Autodesk Inventor part; units mm, degrees
(part 2 of 2)
  spline S217 degree 2 poles (-59.869, -3.174) (-59.9555, -3.2654) (-60.0444, -3.4852) (-60.0567, -3.6309) knots 0 0 0 1 2 2 2
  line L196 (-60.0567, -3.6309) -> (-58.8489, -3.6309)
  line L197 (-54.9784, -5.029) -> (-56.7444, -5.029)
  line L198 (-56.7444, -5.029) -> (-56.7444, -1.981)
  line L199 (-56.7444, -1.981) -> (-56.3394, -1.981)
  line L200 (-56.3394, -1.981) -> (-56.3394, -4.6683)
  line L201 (-56.3394, -4.6683) -> (-54.9784, -4.6683)
  line L202 (-54.9784, -4.6683) -> (-54.9784, -5.029)
  spline S218 degree 2 poles (-53.6964, -5.0808) (-54.2448, -5.0808) (-54.8475, -4.4658) (-54.8475, -3.8977) knots 0 0 0 1 2 2 2
  spline S219 degree 2 poles (-54.8475, -3.8977) (-54.8475, -3.3395) (-54.2621, -2.6775) (-53.7903, -2.6775) knots 0 0 0 1 2 2 2
  spline S220 degree 2 poles (-53.7903, -2.6775) (-53.5779, -2.6775) (-53.2494, -2.801) (-53.1283, -2.9319) knots 0 0 0 1 2 2 2
  spline S221 degree 2 poles (-53.1283, -2.9319) (-53.0048, -3.0628) (-52.8739, -3.4407) (-52.8739, -3.7149) knots 0 0 0 1 2 2 2
  line L203 (-52.8739, -3.7149) -> (-52.8739, -3.9249)
  line L204 (-52.8739, -3.9249) -> (-54.4572, -3.9249)
  spline S222 degree 2 poles (-54.4572, -3.9249) (-54.4572, -4.3225) (-54.0571, -4.7449) (-53.7014, -4.7449) knots 0 0 0 1 2 2 2
  spline S223 degree 2 poles (-53.7014, -4.7449) (-53.5754, -4.7449) (-53.3309, -4.6881) (-53.2321, -4.6436) knots 0 0 0 1 2 2 2
  spline S224 degree 2 poles (-53.2321, -4.6436) (-53.1283, -4.5942) (-52.9851, -4.5078) (-52.9381, -4.4683) knots 0 0 0 1 2 2 2
  line L205 (-52.9381, -4.4683) -> (-52.9159, -4.4683)
  line L206 (-52.9159, -4.4683) -> (-52.9159, -4.8882)
  spline S225 degree 2 poles (-52.9159, -4.8882) (-52.9826, -4.9153) (-53.1851, -4.9944) (-53.2642, -5.0166) knots 0 0 0 1 2 2 2
  spline S226 degree 2 poles (-53.2642, -5.0166) (-53.3753, -5.0487) (-53.5581, -5.0808) (-53.6964, -5.0808) knots 0 0 0 1 2 2 2
  spline S227 degree 2 poles (-53.2494, -3.6309) (-53.2543, -3.4753) (-53.3185, -3.2481) (-53.3803, -3.1715) knots 0 0 0 1 2 2 2
  spline S228 degree 2 poles (-53.3803, -3.1715) (-53.447, -3.085) (-53.6569, -2.9937) (-53.8125, -2.9937) knots 0 0 0 1 2 2 2
  spline S229 degree 2 poles (-53.8125, -2.9937) (-53.9657, -2.9937) (-54.1806, -3.085) (-54.2695, -3.174) knots 0 0 0 1 2 2 2
  spline S230 degree 2 poles (-54.2695, -3.174) (-54.3559, -3.2654) (-54.4449, -3.4852) (-54.4572, -3.6309) knots 0 0 0 1 2 2 2
  line L207 (-54.4572, -3.6309) -> (-53.2494, -3.6309)
  line L208 (-49.8901, -5.029) -> (-49.8901, -3.705)
  spline S231 degree 2 poles (-49.8901, -3.705) (-49.8901, -3.5469) (-49.9148, -3.2777) (-49.9544, -3.2036) knots 0 0 0 1 2 2 2
  spline S232 degree 2 poles (-49.9544, -3.2036) (-49.9939, -3.1221) (-50.1446, -3.0431) (-50.2755, -3.0431) knots 0 0 0 1 2 2 2
  spline S233 degree 2 poles (-50.2755, -3.0431) (-50.394, -3.0431) (-50.6657, -3.1888) (-50.809, -3.3271) knots 0 0 0 1 2 2 2
  spline S234 degree 2 poles (-50.809, -3.3271) (-50.8065, -3.3617) (-50.8016, -3.458) (-50.8016, -3.5222) knots 0 0 0 1 2 2 2
  line L209 (-50.8016, -3.5222) -> (-50.8016, -5.029)
  line L210 (-50.8016, -5.029) -> (-51.1869, -5.029)
  line L211 (-51.1869, -5.029) -> (-51.1869, -3.705)
  spline S235 degree 2 poles (-51.1869, -3.705) (-51.1869, -3.5469) (-51.2116, -3.2777) (-51.2511, -3.2036) knots 0 0 0 1 2 2 2
  spline S236 degree 2 poles (-51.2511, -3.2036) (-51.2906, -3.1221) (-51.4413, -3.0431) (-51.5722, -3.0431) knots 0 0 0 1 2 2 2
  spline S237 degree 2 poles (-51.5722, -3.0431) (-51.6957, -3.0431) (-51.9699, -3.1987) (-52.0983, -3.3197) knots 0 0 0 1 2 2 2
  line L212 (-52.0983, -3.3197) -> (-52.0983, -5.029)
  line L213 (-52.0983, -5.029) -> (-52.4837, -5.029)
  line L214 (-52.4837, -5.029) -> (-52.4837, -2.7417)
  line L215 (-52.4837, -2.7417) -> (-52.0983, -2.7417)
  line L216 (-52.0983, -2.7417) -> (-52.0983, -2.9937)
  spline S238 degree 2 poles (-52.0983, -2.9937) (-51.9477, -2.843) (-51.6513, -2.6775) (-51.4734, -2.6775) knots 0 0 0 1 2 2 2
  spline S239 degree 2 poles (-51.4734, -2.6775) (-51.2709, -2.6775) (-50.9572, -2.8627) (-50.8757, -3.0727) knots 0 0 0 1 2 2 2
  spline S240 degree 2 poles (-50.8757, -3.0727) (-50.7003, -2.8776) (-50.3693, -2.6775) (-50.1767, -2.6775) knots 0 0 0 1 2 2 2
  spline S241 degree 2 poles (-50.1767, -2.6775) (-50.0285, -2.6775) (-49.7864, -2.7689) (-49.6975, -2.8726) knots 0 0 0 1 2 2 2
  spline S242 degree 2 poles (-49.6975, -2.8726) (-49.6061, -2.9764) (-49.5048, -3.2876) (-49.5048, -3.5222) knots 0 0 0 1 2 2 2
  line L217 (-49.5048, -3.5222) -> (-49.5048, -5.029)
  line L218 (-49.5048, -5.029) -> (-49.8901, -5.029)
  spline S243 degree 2 poles (-47.0472, -3.8483) (-47.0472, -4.409) (-47.5906, -5.0932) (-48.0006, -5.0932) knots 0 0 0 1 2 2 2
  spline S244 degree 2 poles (-48.0006, -5.0932) (-48.1858, -5.0932) (-48.4501, -5.0018) (-48.5786, -4.9227) knots 0 0 0 1 2 2 2
  line L219 (-48.5786, -4.9227) -> (-48.6033, -5.029)
  line L220 (-48.6033, -5.029) -> (-48.9639, -5.029)
  line L221 (-48.9639, -5.029) -> (-48.9639, -1.8451)
  line L222 (-48.9639, -1.8451) -> (-48.5786, -1.8451)
  line L223 (-48.5786, -1.8451) -> (-48.5786, -2.9813)
  spline S245 degree 2 poles (-48.5786, -2.9813) (-48.4328, -2.8504) (-48.0944, -2.6775) (-47.8796, -2.6775) knots 0 0 0 1 2 2 2
  spline S246 degree 2 poles (-47.8796, -2.6775) (-47.4918, -2.6775) (-47.0472, -3.2975) (-47.0472, -3.8483) knots 0 0 0 1 2 2 2
  spline S247 degree 2 poles (-47.4448, -3.8779) (-47.4448, -3.4679) (-47.6943, -3.0431) (-47.9709, -3.0431) knots 0 0 0 1 2 2 2
  spline S248 degree 2 poles (-47.9709, -3.0431) (-48.1266, -3.0431) (-48.4477, -3.1913) (-48.5786, -3.3049) knots 0 0 0 1 2 2 2
  line L224 (-48.5786, -3.3049) -> (-48.5786, -4.6165)
  spline S249 degree 2 poles (-48.5786, -4.6165) (-48.4328, -4.6881) (-48.2081, -4.7474) (-48.0747, -4.7474) knots 0 0 0 1 2 2 2
  spline S250 degree 2 poles (-48.0747, -4.7474) (-47.7808, -4.7474) (-47.4448, -4.3299) (-47.4448, -3.8779) knots 0 0 0 1 2 2 2
  spline S251 degree 2 poles (-44.7673, -3.8853) (-44.7673, -4.4633) (-45.3231, -5.0932) (-45.7874, -5.0932) knots 0 0 0 1 2 2 2
  spline S252 degree 2 poles (-45.7874, -5.0932) (-46.2642, -5.0932) (-46.81, -4.4436) (-46.81, -3.8853) knots 0 0 0 1 2 2 2
  spline S253 degree 2 poles (-46.81, -3.8853) (-46.81, -3.3123) (-46.2469, -2.6775) (-45.7874, -2.6775) knots 0 0 0 1 2 2 2
  spline S254 degree 2 poles (-45.7874, -2.6775) (-45.3231, -2.6775) (-44.7673, -3.3098) (-44.7673, -3.8853) knots 0 0 0 1 2 2 2
  spline S255 degree 2 poles (-45.165, -3.8853) (-45.165, -3.4407) (-45.4886, -3.0085) (-45.7874, -3.0085) knots 0 0 0 1 2 2 2
  spline S256 degree 2 poles (-45.7874, -3.0085) (-46.0863, -3.0085) (-46.4124, -3.4407) (-46.4124, -3.8853) knots 0 0 0 1 2 2 2
  spline S257 degree 2 poles (-46.4124, -3.8853) (-46.4124, -4.3176) (-46.0863, -4.7622) (-45.7874, -4.7622) knots 0 0 0 1 2 2 2
  spline S258 degree 2 poles (-45.7874, -4.7622) (-45.491, -4.7622) (-45.165, -4.325) (-45.165, -3.8853) knots 0 0 0 1 2 2 2
  line L225 (-42.0034, -3.8804) -> (-43.1569, -3.8804)
  line L226 (-43.1569, -3.8804) -> (-43.1569, -3.5099)
  line L227 (-43.1569, -3.5099) -> (-42.0034, -3.5099)
  line L228 (-42.0034, -3.5099) -> (-42.0034, -3.8804)
  line L229 (-39.4914, -5.029) -> (-39.4914, -2.3416)
  line L230 (-39.4914, -2.3416) -> (-40.514, -2.3416)
  line L231 (-40.514, -2.3416) -> (-40.514, -1.981)
  line L232 (-40.514, -1.981) -> (-38.0637, -1.981)
  line L233 (-38.0637, -1.981) -> (-38.0637, -2.3416)
  line L234 (-38.0637, -2.3416) -> (-39.0863, -2.3416)
  line L235 (-39.0863, -2.3416) -> (-39.0863, -5.029)
  line L236 (-39.0863, -5.029) -> (-39.4914, -5.029)
  spline S259 degree 2 poles (-35.9049, -3.8853) (-35.9049, -4.4633) (-36.4607, -5.0932) (-36.925, -5.0932) knots 0 0 0 1 2 2 2
  spline S260 degree 2 poles (-36.925, -5.0932) (-37.4017, -5.0932) (-37.9476, -4.4436) (-37.9476, -3.8853) knots 0 0 0 1 2 2 2
  spline S261 degree 2 poles (-37.9476, -3.8853) (-37.9476, -3.3123) (-37.3845, -2.6775) (-36.925, -2.6775) knots 0 0 0 1 2 2 2
  spline S262 degree 2 poles (-36.925, -2.6775) (-36.4607, -2.6775) (-35.9049, -3.3098) (-35.9049, -3.8853) knots 0 0 0 1 2 2 2
  spline S263 degree 2 poles (-36.3026, -3.8853) (-36.3026, -3.4407) (-36.6262, -3.0085) (-36.925, -3.0085) knots 0 0 0 1 2 2 2
  spline S264 degree 2 poles (-36.925, -3.0085) (-37.2239, -3.0085) (-37.5499, -3.4407) (-37.5499, -3.8853) knots 0 0 0 1 2 2 2
  spline S265 degree 2 poles (-37.5499, -3.8853) (-37.5499, -4.3176) (-37.2239, -4.7622) (-36.925, -4.7622) knots 0 0 0 1 2 2 2
  spline S266 degree 2 poles (-36.925, -4.7622) (-36.6286, -4.7622) (-36.3026, -4.325) (-36.3026, -3.8853) knots 0 0 0 1 2 2 2
  line L237 (-32.9162, -5.029) -> (-32.9162, -3.705)
  spline S267 degree 2 poles (-32.9162, -3.705) (-32.9162, -3.5469) (-32.9409, -3.2777) (-32.9804, -3.2036) knots 0 0 0 1 2 2 2
  spline S268 degree 2 poles (-32.9804, -3.2036) (-33.0199, -3.1221) (-33.1706, -3.0431) (-33.3015, -3.0431) knots 0 0 0 1 2 2 2
  spline S269 degree 2 poles (-33.3015, -3.0431) (-33.4201, -3.0431) (-33.6918, -3.1888) (-33.835, -3.3271) knots 0 0 0 1 2 2 2
  spline S270 degree 2 poles (-33.835, -3.3271) (-33.8326, -3.3617) (-33.8276, -3.458) (-33.8276, -3.5222) knots 0 0 0 1 2 2 2
  line L238 (-33.8276, -3.5222) -> (-33.8276, -5.029)
  line L239 (-33.8276, -5.029) -> (-34.213, -5.029)
  line L240 (-34.213, -5.029) -> (-34.213, -3.705)
  spline S271 degree 2 poles (-34.213, -3.705) (-34.213, -3.5469) (-34.2377, -3.2777) (-34.2772, -3.2036) knots 0 0 0 1 2 2 2
  spline S272 degree 2 poles (-34.2772, -3.2036) (-34.3167, -3.1221) (-34.4674, -3.0431) (-34.5983, -3.0431) knots 0 0 0 1 2 2 2
  spline S273 degree 2 poles (-34.5983, -3.0431) (-34.7218, -3.0431) (-34.9959, -3.1987) (-35.1244, -3.3197) knots 0 0 0 1 2 2 2
  line L241 (-35.1244, -3.3197) -> (-35.1244, -5.029)
  line L242 (-35.1244, -5.029) -> (-35.5097, -5.029)
  line L243 (-35.5097, -5.029) -> (-35.5097, -2.7417)
  line L244 (-35.5097, -2.7417) -> (-35.1244, -2.7417)
  line L245 (-35.1244, -2.7417) -> (-35.1244, -2.9937)
  spline S274 degree 2 poles (-35.1244, -2.9937) (-34.9737, -2.843) (-34.6773, -2.6775) (-34.4995, -2.6775) knots 0 0 0 1 2 2 2
  spline S275 degree 2 poles (-34.4995, -2.6775) (-34.2969, -2.6775) (-33.9832, -2.8627) (-33.9017, -3.0727) knots 0 0 0 1 2 2 2
  spline S276 degree 2 poles (-33.9017, -3.0727) (-33.7264, -2.8776) (-33.3954, -2.6775) (-33.2027, -2.6775) knots 0 0 0 1 2 2 2
  spline S277 degree 2 poles (-33.2027, -2.6775) (-33.0545, -2.6775) (-32.8125, -2.7689) (-32.7235, -2.8726) knots 0 0 0 1 2 2 2
  spline S278 degree 2 poles (-32.7235, -2.8726) (-32.6321, -2.9764) (-32.5309, -3.2876) (-32.5309, -3.5222) knots 0 0 0 1 2 2 2
  line L246 (-32.5309, -3.5222) -> (-32.5309, -5.029)
  line L247 (-32.5309, -5.029) -> (-32.9162, -5.029)
  spline S279 degree 2 poles (-28.7246, -2.8998) (-28.7246, -3.0974) (-28.8654, -3.4531) (-28.9913, -3.5766) knots 0 0 0 1 2 2 2
  spline S280 degree 2 poles (-28.9913, -3.5766) (-29.1494, -3.7322) (-29.5767, -3.8927) (-29.9028, -3.8927) knots 0 0 0 1 2 2 2
  line L248 (-29.9028, -3.8927) -> (-30.2461, -3.8927)
  line L249 (-30.2461, -3.8927) -> (-30.2461, -5.029)
  line L250 (-30.2461, -5.029) -> (-30.6512, -5.029)
  line L251 (-30.6512, -5.029) -> (-30.6512, -1.981)
  line L252 (-30.6512, -1.981) -> (-29.8855, -1.981)
  spline S281 degree 2 poles (-29.8855, -1.981) (-29.6138, -1.981) (-29.2334, -2.0699) (-29.0877, -2.1711) knots 0 0 0 1 2 2 2
  spline S282 degree 2 poles (-29.0877, -2.1711) (-28.9172, -2.2872) (-28.7246, -2.6454) (-28.7246, -2.8998) knots 0 0 0 1 2 2 2
  spline S283 degree 2 poles (-29.1469, -2.9121) (-29.1469, -2.7541) (-29.2556, -2.5219) (-29.3668, -2.4478) knots 0 0 0 1 2 2 2
  spline S284 degree 2 poles (-29.3668, -2.4478) (-29.4631, -2.3836) (-29.72, -2.3317) (-29.9102, -2.3317) knots 0 0 0 1 2 2 2
  line L253 (-29.9102, -2.3317) -> (-30.2461, -2.3317)
  line L254 (-30.2461, -2.3317) -> (-30.2461, -3.5469)
  line L255 (-30.2461, -3.5469) -> (-29.9695, -3.5469)
  spline S285 degree 2 poles (-29.9695, -3.5469) (-29.7225, -3.5469) (-29.4187, -3.4679) (-29.3199, -3.3642) knots 0 0 0 1 2 2 2
  spline S286 degree 2 poles (-29.3199, -3.3642) (-29.2285, -3.2728) (-29.1469, -3.0579) (-29.1469, -2.9121) knots 0 0 0 1 2 2 2
  line L256 (-27.166, -2.2156) -> (-27.1858, -2.2156)
  spline S287 degree 2 poles (-27.1858, -2.2156) (-27.2376, -2.1958) (-27.4303, -2.1613) (-27.5069, -2.1613) knots 0 0 0 1 2 2 2
  spline S288 degree 2 poles (-27.5069, -2.1613) (-27.7489, -2.1613) (-27.9564, -2.3786) (-27.9564, -2.6651) knots 0 0 0 1 2 2 2
  line L257 (-27.9564, -2.6651) -> (-27.9564, -2.7417)
  line L258 (-27.9564, -2.7417) -> (-27.3191, -2.7417)
  line L259 (-27.3191, -2.7417) -> (-27.3191, -3.0603)
  line L260 (-27.3191, -3.0603) -> (-27.9441, -3.0603)
  line L261 (-27.9441, -3.0603) -> (-27.9441, -5.029)
  line L262 (-27.9441, -5.029) -> (-28.3294, -5.029)
  line L263 (-28.3294, -5.029) -> (-28.3294, -3.0603)
  line L264 (-28.3294, -3.0603) -> (-28.5887, -3.0603)
  line L265 (-28.5887, -3.0603) -> (-28.5887, -2.7417)
  line L266 (-28.5887, -2.7417) -> (-28.3294, -2.7417)
  line L267 (-28.3294, -2.7417) -> (-28.3294, -2.6651)
  spline S289 degree 2 poles (-28.3294, -2.6651) (-28.3294, -2.2551) (-27.9317, -1.8253) (-27.5612, -1.8253) knots 0 0 0 1 2 2 2
  spline S290 degree 2 poles (-27.5612, -1.8253) (-27.455, -1.8253) (-27.25, -1.8476) (-27.166, -1.8624) knots 0 0 0 1 2 2 2
  line L268 (-27.166, -1.8624) -> (-27.166, -2.2156)
  spline S291 degree 2 poles (-25.7606, -4.7869) (-25.8075, -4.8215) (-25.9656, -4.945) (-26.0397, -4.982) knots 0 0 0 1 2 2 2
  spline S292 degree 2 poles (-26.0397, -4.982) (-26.1409, -5.0364) (-26.3311, -5.0932) (-26.504, -5.0932) knots 0 0 0 1 2 2 2
  spline S293 degree 2 poles (-26.504, -5.0932) (-26.6448, -5.0932) (-26.8992, -4.987) (-26.9956, -4.8906) knots 0 0 0 1 2 2 2
  spline S294 degree 2 poles (-26.9956, -4.8906) (-27.087, -4.7968) (-27.1981, -4.5201) (-27.1981, -4.367) knots 0 0 0 1 2 2 2
  spline S295 degree 2 poles (-27.1981, -4.367) (-27.1981, -4.1299) (-26.998, -3.7939) (-26.7807, -3.6976) knots 0 0 0 1 2 2 2
  spline S296 degree 2 poles (-26.7807, -3.6976) (-26.588, -3.6087) (-26.0644, -3.542) (-25.7606, -3.5247) knots 0 0 0 1 2 2 2
  line L269 (-25.7606, -3.5247) -> (-25.7606, -3.4506)
  spline S297 degree 2 poles (-25.7606, -3.4506) (-25.7606, -3.3172) (-25.8421, -3.1517) (-25.9162, -3.1048) knots 0 0 0 1 2 2 2
  spline S298 degree 2 poles (-25.9162, -3.1048) (-25.9903, -3.0579) (-26.2027, -3.0282) (-26.3163, -3.0282) knots 0 0 0 1 2 2 2
  spline S299 degree 2 poles (-26.3163, -3.0282) (-26.4497, -3.0282) (-26.8103, -3.1073) (-26.9906, -3.1838) knots 0 0 0 1 2 2 2
  line L270 (-26.9906, -3.1838) -> (-27.0129, -3.1838)
  line L271 (-27.0129, -3.1838) -> (-27.0129, -2.7911)
  spline S300 degree 2 poles (-27.0129, -2.7911) (-26.9066, -2.7615) (-26.509, -2.6874) (-26.3138, -2.6874) knots 0 0 0 1 2 2 2
  spline S301 degree 2 poles (-26.3138, -2.6874) (-26.0767, -2.6874) (-25.7531, -2.7615) (-25.6247, -2.8578) knots 0 0 0 1 2 2 2
  spline S302 degree 2 poles (-25.6247, -2.8578) (-25.4987, -2.9517) (-25.3752, -3.2505) (-25.3752, -3.4654) knots 0 0 0 1 2 2 2
  line L272 (-25.3752, -3.4654) -> (-25.3752, -5.029)
  line L273 (-25.3752, -5.029) -> (-25.7606, -5.029)
  line L274 (-25.7606, -5.029) -> (-25.7606, -4.7869)
  line L275 (-25.7606, -4.4658) -> (-25.7606, -3.831)
  spline S303 degree 2 poles (-25.7606, -3.831) (-25.8989, -3.8433) (-26.3163, -3.8853) (-26.4472, -3.9249) knots 0 0 0 1 2 2 2
  spline S304 degree 2 poles (-26.4472, -3.9249) (-26.6004, -3.9718) (-26.8004, -4.1669) (-26.8004, -4.3398) knots 0 0 0 1 2 2 2
  spline S305 degree 2 poles (-26.8004, -4.3398) (-26.8004, -4.5374) (-26.5781, -4.7375) (-26.3657, -4.7375) knots 0 0 0 1 2 2 2
  spline S306 degree 2 poles (-26.3657, -4.7375) (-26.1854, -4.7375) (-25.889, -4.5819) (-25.7606, -4.4658) knots 0 0 0 1 2 2 2
  line L276 (-23.6314, -2.2156) -> (-23.6512, -2.2156)
  spline S307 degree 2 poles (-23.6512, -2.2156) (-23.703, -2.1958) (-23.8957, -2.1613) (-23.9723, -2.1613) knots 0 0 0 1 2 2 2
  spline S308 degree 2 poles (-23.9723, -2.1613) (-24.2143, -2.1613) (-24.4218, -2.3786) (-24.4218, -2.6651) knots 0 0 0 1 2 2 2
  line L277 (-24.4218, -2.6651) -> (-24.4218, -2.7417)
  line L278 (-24.4218, -2.7417) -> (-23.7845, -2.7417)
  line L279 (-23.7845, -2.7417) -> (-23.7845, -3.0603)
  line L280 (-23.7845, -3.0603) -> (-24.4095, -3.0603)
  line L281 (-24.4095, -3.0603) -> (-24.4095, -5.029)
  line L282 (-24.4095, -5.029) -> (-24.7948, -5.029)
  line L283 (-24.7948, -5.029) -> (-24.7948, -3.0603)
  line L284 (-24.7948, -3.0603) -> (-25.0541, -3.0603)
  line L285 (-25.0541, -3.0603) -> (-25.0541, -2.7417)
  line L286 (-25.0541, -2.7417) -> (-24.7948, -2.7417)
  line L287 (-24.7948, -2.7417) -> (-24.7948, -2.6651)
  spline S309 degree 2 poles (-24.7948, -2.6651) (-24.7948, -2.2551) (-24.3971, -1.8253) (-24.0266, -1.8253) knots 0 0 0 1 2 2 2
  spline S310 degree 2 poles (-24.0266, -1.8253) (-23.9204, -1.8253) (-23.7154, -1.8476) (-23.6314, -1.8624) knots 0 0 0 1 2 2 2
  line L288 (-23.6314, -1.8624) -> (-23.6314, -2.2156)
  line L289 (-22.2976, -2.2156) -> (-22.3174, -2.2156)
  spline S311 degree 2 poles (-22.3174, -2.2156) (-22.3692, -2.1958) (-22.5619, -2.1613) (-22.6385, -2.1613) knots 0 0 0 1 2 2 2
  spline S312 degree 2 poles (-22.6385, -2.1613) (-22.8805, -2.1613) (-23.088, -2.3786) (-23.088, -2.6651) knots 0 0 0 1 2 2 2
  line L290 (-23.088, -2.6651) -> (-23.088, -2.7417)
  line L291 (-23.088, -2.7417) -> (-22.4507, -2.7417)
  line L292 (-22.4507, -2.7417) -> (-22.4507, -3.0603)
  line L293 (-22.4507, -3.0603) -> (-23.0756, -3.0603)
  line L294 (-23.0756, -3.0603) -> (-23.0756, -5.029)
  line L295 (-23.0756, -5.029) -> (-23.461, -5.029)
  line L296 (-23.461, -5.029) -> (-23.461, -3.0603)
  line L297 (-23.461, -3.0603) -> (-23.7203, -3.0603)
  line L298 (-23.7203, -3.0603) -> (-23.7203, -2.7417)
  line L299 (-23.7203, -2.7417) -> (-23.461, -2.7417)
  line L300 (-23.461, -2.7417) -> (-23.461, -2.6651)
  spline S313 degree 2 poles (-23.461, -2.6651) (-23.461, -2.2551) (-23.0633, -1.8253) (-22.6928, -1.8253) knots 0 0 0 1 2 2 2
  spline S314 degree 2 poles (-22.6928, -1.8253) (-22.5866, -1.8253) (-22.3816, -1.8476) (-22.2976, -1.8624) knots 0 0 0 1 2 2 2
  line L301 (-22.2976, -1.8624) -> (-22.2976, -2.2156)
  spline S315 degree 2 poles (-21.1737, -5.0808) (-21.7221, -5.0808) (-22.3248, -4.4658) (-22.3248, -3.8977) knots 0 0 0 1 2 2 2
  spline S316 degree 2 poles (-22.3248, -3.8977) (-22.3248, -3.3395) (-21.7394, -2.6775) (-21.2676, -2.6775) knots 0 0 0 1 2 2 2
  spline S317 degree 2 poles (-21.2676, -2.6775) (-21.0552, -2.6775) (-20.7267, -2.801) (-20.6056, -2.9319) knots 0 0 0 1 2 2 2
  spline S318 degree 2 poles (-20.6056, -2.9319) (-20.4821, -3.0628) (-20.3512, -3.4407) (-20.3512, -3.7149) knots 0 0 0 1 2 2 2
  line L302 (-20.3512, -3.7149) -> (-20.3512, -3.9249)
  line L303 (-20.3512, -3.9249) -> (-21.9345, -3.9249)
  spline S319 degree 2 poles (-21.9345, -3.9249) (-21.9345, -4.3225) (-21.5344, -4.7449) (-21.1787, -4.7449) knots 0 0 0 1 2 2 2
  spline S320 degree 2 poles (-21.1787, -4.7449) (-21.0527, -4.7449) (-20.8082, -4.6881) (-20.7094, -4.6436) knots 0 0 0 1 2 2 2
  spline S321 degree 2 poles (-20.7094, -4.6436) (-20.6056, -4.5942) (-20.4624, -4.5078) (-20.4154, -4.4683) knots 0 0 0 1 2 2 2
  line L304 (-20.4154, -4.4683) -> (-20.3932, -4.4683)
  line L305 (-20.3932, -4.4683) -> (-20.3932, -4.8882)
  spline S322 degree 2 poles (-20.3932, -4.8882) (-20.4599, -4.9153) (-20.6624, -4.9944) (-20.7415, -5.0166) knots 0 0 0 1 2 2 2
  spline S323 degree 2 poles (-20.7415, -5.0166) (-20.8526, -5.0487) (-21.0354, -5.0808) (-21.1737, -5.0808) knots 0 0 0 1 2 2 2
  spline S324 degree 2 poles (-20.7267, -3.6309) (-20.7316, -3.4753) (-20.7958, -3.2481) (-20.8576, -3.1715) knots 0 0 0 1 2 2 2
  spline S325 degree 2 poles (-20.8576, -3.1715) (-20.9243, -3.085) (-21.1342, -2.9937) (-21.2898, -2.9937) knots 0 0 0 1 2 2 2
  spline S326 degree 2 poles (-21.2898, -2.9937) (-21.443, -2.9937) (-21.6579, -3.085) (-21.7468, -3.174) knots 0 0 0 1 2 2 2
  spline S327 degree 2 poles (-21.7468, -3.174) (-21.8332, -3.2654) (-21.9222, -3.4852) (-21.9345, -3.6309) knots 0 0 0 1 2 2 2
  line L306 (-21.9345, -3.6309) -> (-20.7267, -3.6309)
  spline S328 degree 2 poles (-62.8907, 59.8443) (-62.4491, 59.8443) (-61.7927, 59.6133) (-61.5617, 59.3824) knots 0 0 0 1 2 2 2
  spline S329 degree 2 poles (-61.5617, 59.3824) (-61.2984, 59.1231) (-61.0836, 58.3937) (-61.0836, 57.8589) knots 0 0 0 1 2 2 2
  line L307 (-61.0836, 57.8589) -> (-61.0836, 54.7389)
  line L308 (-61.0836, 54.7389) -> (-61.7481, 54.7389)
  line L309 (-61.7481, 54.7389) -> (-61.7481, 57.8589)
  spline S330 degree 2 poles (-61.7481, 57.8589) (-61.7481, 58.2073) (-61.8373, 58.6774) (-61.9629, 58.8678) knots 0 0 0 1 2 2 2
  spline S331 degree 2 poles (-61.9629, 58.8678) (-62.0966, 59.0704) (-62.5585, 59.277) (-62.8907, 59.277) knots 0 0 0 1 2 2 2
  spline S332 degree 2 poles (-62.8907, 59.277) (-63.2027, 59.277) (-63.689, 59.0704) (-63.8227, 58.8678) knots 0 0 0 1 2 2 2
  spline S333 degree 2 poles (-63.8227, 58.8678) (-63.9483, 58.6774) (-64.0374, 58.2114) (-64.0374, 57.8751) knots 0 0 0 1 2 2 2
  line L310 (-64.0374, 57.8751) -> (-64.0374, 54.7389)
  line L311 (-64.0374, 54.7389) -> (-64.7019, 54.7389)
  line L312 (-64.7019, 54.7389) -> (-64.7019, 57.8589)
  spline S334 degree 2 poles (-64.7019, 57.8589) (-64.7019, 58.3816) (-64.4912, 59.1271) (-64.2238, 59.3824) knots 0 0 0 1 2 2 2
  spline S335 degree 2 poles (-64.2238, 59.3824) (-63.9847, 59.6174) (-63.3527, 59.8443) (-62.8907, 59.8443) knots 0 0 0 1 2 2 2
  spline S336 degree 2 poles (-69.0455, 58.2033) (-69.0455, 58.5761) (-68.7619, 59.1474) (-68.5269, 59.3338) knots 0 0 0 1 2 2 2
  spline S337 degree 2 poles (-68.5269, 59.3338) (-68.2433, 59.5526) (-67.599, 59.7389) (-67.0885, 59.7389) knots 0 0 0 1 2 2 2
  line L313 (-67.0885, 59.7389) -> (-65.6541, 59.7389)
  line L314 (-65.6541, 59.7389) -> (-65.6541, 54.7389)
  line L315 (-65.6541, 54.7389) -> (-66.9791, 54.7389)
  spline S338 degree 2 poles (-66.9791, 54.7389) (-67.5139, 54.7389) (-68.0488, 54.8078) (-68.2919, 54.9415) knots 0 0 0 1 2 2 2
  spline S339 degree 2 poles (-68.2919, 54.9415) (-68.5634, 55.0834) (-68.8105, 55.5493) (-68.8105, 55.8654) knots 0 0 0 1 2 2 2
  spline S340 degree 2 poles (-68.8105, 55.8654) (-68.8105, 56.2179) (-68.4377, 56.777) (-68.1095, 56.9351) knots 0 0 0 1 2 2 2
  line L316 (-68.1095, 56.9351) -> (-68.1095, 56.9594)
  spline S341 degree 2 poles (-68.1095, 56.9594) (-68.5553, 57.0809) (-69.0455, 57.7252) (-69.0455, 58.2033) knots 0 0 0 1 2 2 2
  spline S342 degree 2 poles (-68.3527, 58.2316) (-68.3527, 57.948) (-68.1906, 57.5834) (-67.9475, 57.4537) knots 0 0 0 1 2 2 2
  spline S343 degree 2 poles (-67.9475, 57.4537) (-67.7894, 57.3727) (-67.4167, 57.324) (-67.0723, 57.324) knots 0 0 0 1 2 2 2
  line L317 (-67.0723, 57.324) -> (-66.3186, 57.324)
  line L318 (-66.3186, 57.324) -> (-66.3186, 59.1717)
  line L319 (-66.3186, 59.1717) -> (-66.8575, 59.1717)
  spline S344 degree 2 poles (-66.8575, 59.1717) (-67.2951, 59.1717) (-67.7976, 59.0906) (-67.992, 58.961) knots 0 0 0 1 2 2 2
  spline S345 degree 2 poles (-67.992, 58.961) (-68.1784, 58.8273) (-68.3527, 58.495) (-68.3527, 58.2316) knots 0 0 0 1 2 2 2
  spline S346 degree 2 poles (-68.1176, 55.9586) (-68.1176, 55.7803) (-67.9961, 55.5128) (-67.8624, 55.4359) knots 0 0 0 1 2 2 2
  spline S347 degree 2 poles (-67.8624, 55.4359) (-67.7003, 55.3467) (-67.3073, 55.3062) (-66.9548, 55.3062) knots 0 0 0 1 2 2 2
  line L320 (-66.9548, 55.3062) -> (-66.3186, 55.3062)
  line L321 (-66.3186, 55.3062) -> (-66.3186, 56.7689)
  line L322 (-66.3186, 56.7689) -> (-67.0723, 56.7689)
  spline S348 degree 2 poles (-67.0723, 56.7689) (-67.3843, 56.7689) (-67.68, 56.7041) (-67.8381, 56.6028) knots 0 0 0 1 2 2 2
  spline S349 degree 2 poles (-67.8381, 56.6028) (-67.992, 56.5056) (-68.1176, 56.1936) (-68.1176, 55.9586) knots 0 0 0 1 2 2 2
  spline S350 degree 2 poles (-73.2473, 59.8281) (-72.7044, 59.8281) (-71.9426, 59.6012) (-71.6063, 59.4391) knots 0 0 0 1 2 2 2
  line L323 (-71.6063, 59.4391) -> (-71.6063, 58.6044)
  line L324 (-71.6063, 58.6044) -> (-71.6549, 58.6044)
  spline S351 degree 2 poles (-71.6549, 58.6044) (-71.9831, 58.9124) (-72.8138, 59.2527) (-73.1987, 59.2527) knots 0 0 0 1 2 2 2
  spline S352 degree 2 poles (-73.1987, 59.2527) (-73.7497, 59.2527) (-74.3129, 58.7949) (-74.3129, 58.418) knots 0 0 0 1 2 2 2
  spline S353 degree 2 poles (-74.3129, 58.418) (-74.3129, 58.1182) (-74.0172, 57.7454) (-73.6971, 57.6522) knots 0 0 0 1 2 2 2
  spline S354 degree 2 poles (-73.6971, 57.6522) (-73.4661, 57.5874) (-73.0812, 57.4983) (-72.7935, 57.4253) knots 0 0 0 1 2 2 2
  spline S355 degree 2 poles (-72.7935, 57.4253) (-72.5342, 57.3564) (-72.1249, 57.1498) (-71.9669, 56.9837) knots 0 0 0 1 2 2 2
  spline S356 degree 2 poles (-71.9669, 56.9837) (-71.8129, 56.8175) (-71.6428, 56.3718) (-71.6428, 56.0801) knots 0 0 0 1 2 2 2
  spline S357 degree 2 poles (-71.6428, 56.0801) (-71.6428, 55.4723) (-72.5909, 54.6498) (-73.3243, 54.6498) knots 0 0 0 1 2 2 2
  spline S358 degree 2 poles (-73.3243, 54.6498) (-73.7457, 54.6498) (-74.4912, 54.8159) (-74.8113, 54.974) knots 0 0 0 1 2 2 2
  line L325 (-74.8113, 54.974) -> (-74.8113, 55.7681)
  line L326 (-74.8113, 55.7681) -> (-74.7627, 55.7681)
  spline S359 degree 2 poles (-74.7627, 55.7681) (-74.5236, 55.5493) (-73.7781, 55.2252) (-73.3689, 55.2252) knots 0 0 0 1 2 2 2
  spline S360 degree 2 poles (-73.3689, 55.2252) (-72.907, 55.2252) (-72.3356, 55.6587) (-72.3356, 56.0112) knots 0 0 0 1 2 2 2
  spline S361 degree 2 poles (-72.3356, 56.0112) (-72.3356, 56.3273) (-72.6719, 56.7041) (-72.988, 56.7892) knots 0 0 0 1 2 2 2
  spline S362 degree 2 poles (-72.988, 56.7892) (-73.1987, 56.8459) (-73.8105, 56.9918) (-74.0131, 57.0526) knots 0 0 0 1 2 2 2
  spline S363 degree 2 poles (-74.0131, 57.0526) (-74.5277, 57.2106) (-75.0058, 57.8467) (-75.0058, 58.3127) knots 0 0 0 1 2 2 2
  spline S364 degree 2 poles (-75.0058, 58.3127) (-75.0058, 58.6085) (-74.7668, 59.1757) (-74.552, 59.3743) knots 0 0 0 1 2 2 2
  spline S365 degree 2 poles (-74.552, 59.3743) (-74.3129, 59.5931) (-73.7052, 59.8281) (-73.2473, 59.8281) knots 0 0 0 1 2 2 2
  line L327 (-75.6825, 59.7389) -> (-75.6825, 54.7389)
  line L328 (-75.6825, 54.7389) -> (-78.8105, 54.7389)
  line L329 (-78.8105, 54.7389) -> (-78.8105, 55.3305)
  line L330 (-78.8105, 55.3305) -> (-76.347, 55.3305)
  line L331 (-76.347, 55.3305) -> (-76.347, 56.7)
  line L332 (-76.347, 56.7) -> (-78.6444, 56.7)
  line L333 (-78.6444, 56.7) -> (-78.6444, 57.2916)
  line L334 (-78.6444, 57.2916) -> (-76.347, 57.2916)
  line L335 (-76.347, 57.2916) -> (-76.347, 59.1474)
  line L336 (-76.347, 59.1474) -> (-78.8105, 59.1474)
  line L337 (-78.8105, 59.1474) -> (-78.8105, 59.7389)
  line L338 (-78.8105, 59.7389) -> (-75.6825, 59.7389)
  spline S366 degree 2 poles (-83.4823, 57.243) (-83.4823, 57.9278) (-82.9272, 59.0299) (-82.4612, 59.3378) knots 0 0 0 1 2 2 2
  spline S367 degree 2 poles (-82.4612, 59.3378) (-82.0804, 59.5769) (-81.2984, 59.7389) (-80.6906, 59.7389) knots 0 0 0 1 2 2 2
  line L339 (-80.6906, 59.7389) -> (-79.5399, 59.7389)
  line L340 (-79.5399, 59.7389) -> (-79.5399, 54.7389)
  line L341 (-79.5399, 54.7389) -> (-80.6784, 54.7389)
  spline S368 degree 2 poles (-80.6784, 54.7389) (-81.3835, 54.7389) (-82.1857, 54.9496) (-82.4694, 55.136) knots 0 0 0 1 2 2 2
  spline S369 degree 2 poles (-82.4694, 55.136) (-82.9515, 55.4561) (-83.4823, 56.5137) (-83.4823, 57.243) knots 0 0 0 1 2 2 2
  spline S370 degree 2 poles (-82.7894, 57.2349) (-82.7894, 56.6595) (-82.4086, 55.8451) (-82.0317, 55.6141) knots 0 0 0 1 2 2 2
  spline S371 degree 2 poles (-82.0317, 55.6141) (-81.7643, 55.4561) (-81.1606, 55.3143) (-80.7108, 55.3143) knots 0 0 0 1 2 2 2
  line L342 (-80.7108, 55.3143) -> (-80.2044, 55.3143)
  line L343 (-80.2044, 55.3143) -> (-80.2044, 59.1636)
  line L344 (-80.2044, 59.1636) -> (-80.7108, 59.1636)
  spline S372 degree 2 poles (-80.7108, 59.1636) (-81.1525, 59.1636) (-81.8211, 59.0218) (-82.0925, 58.8313) knots 0 0 0 1 2 2 2
  spline S373 degree 2 poles (-82.0925, 58.8313) (-82.441, 58.5963) (-82.7894, 57.8184) (-82.7894, 57.2349) knots 0 0 0 1 2 2 2
  spline S374 degree 2 poles (-85.5974, 59.8281) (-85.0544, 59.8281) (-84.2927, 59.6012) (-83.9564, 59.4391) knots 0 0 0 1 2 2 2
  line L345 (-83.9564, 59.4391) -> (-83.9564, 58.6044)
  line L346 (-83.9564, 58.6044) -> (-84.005, 58.6044)
  spline S375 degree 2 poles (-84.005, 58.6044) (-84.3332, 58.9124) (-85.1638, 59.2527) (-85.5488, 59.2527) knots 0 0 0 1 2 2 2
  spline S376 degree 2 poles (-85.5488, 59.2527) (-86.0998, 59.2527) (-86.663, 58.7949) (-86.663, 58.418) knots 0 0 0 1 2 2 2
  spline S377 degree 2 poles (-86.663, 58.418) (-86.663, 58.1182) (-86.3672, 57.7454) (-86.0471, 57.6522) knots 0 0 0 1 2 2 2
  spline S378 degree 2 poles (-86.0471, 57.6522) (-85.8162, 57.5874) (-85.4313, 57.4983) (-85.1436, 57.4253) knots 0 0 0 1 2 2 2
  spline S379 degree 2 poles (-85.1436, 57.4253) (-84.8843, 57.3564) (-84.475, 57.1498) (-84.317, 56.9837) knots 0 0 0 1 2 2 2
  spline S380 degree 2 poles (-84.317, 56.9837) (-84.163, 56.8175) (-83.9929, 56.3718) (-83.9929, 56.0801) knots 0 0 0 1 2 2 2
  spline S381 degree 2 poles (-83.9929, 56.0801) (-83.9929, 55.4723) (-84.941, 54.6498) (-85.6744, 54.6498) knots 0 0 0 1 2 2 2
  spline S382 degree 2 poles (-85.6744, 54.6498) (-86.0958, 54.6498) (-86.8413, 54.8159) (-87.1614, 54.974) knots 0 0 0 1 2 2 2
  line L347 (-87.1614, 54.974) -> (-87.1614, 55.7681)
  line L348 (-87.1614, 55.7681) -> (-87.1128, 55.7681)
  spline S383 degree 2 poles (-87.1128, 55.7681) (-86.8737, 55.5493) (-86.1282, 55.2252) (-85.7189, 55.2252) knots 0 0 0 1 2 2 2
  spline S384 degree 2 poles (-85.7189, 55.2252) (-85.257, 55.2252) (-84.6857, 55.6587) (-84.6857, 56.0112) knots 0 0 0 1 2 2 2
  spline S385 degree 2 poles (-84.6857, 56.0112) (-84.6857, 56.3273) (-85.022, 56.7041) (-85.3381, 56.7892) knots 0 0 0 1 2 2 2
  spline S386 degree 2 poles (-85.3381, 56.7892) (-85.5488, 56.8459) (-86.1606, 56.9918) (-86.3632, 57.0526) knots 0 0 0 1 2 2 2
  spline S387 degree 2 poles (-86.3632, 57.0526) (-86.8778, 57.2106) (-87.3559, 57.8467) (-87.3559, 58.3127) knots 0 0 0 1 2 2 2
  spline S388 degree 2 poles (-87.3559, 58.3127) (-87.3559, 58.6085) (-87.1168, 59.1757) (-86.9021, 59.3743) knots 0 0 0 1 2 2 2
  spline S389 degree 2 poles (-86.9021, 59.3743) (-86.663, 59.5931) (-86.0553, 59.8281) (-85.5974, 59.8281) knots 0 0 0 1 2 2 2
  point P0 (0, 0)
  dimension "d102" = 3
  dimension "d103" = 270
  dimension "d104" = 3
  constraints: 4 other
  measures "d102" distance between parallel lines of L4 L2
  measures "d104" distance from line of L9.start L7
extrude "Extrusion11" cut sketch "Sketch13" against normal blind 1
body "Solid1"
